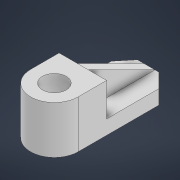
# Autodesk Inventor part: Pieza de práctica 4
Saved by Autodesk Inventor 2022 (Build 260153000, 153)
## iProperties
Created: 2022-06-27
Part Number: Pieza de práctica 4
Material: Genérico
Document SubType Name: Modeling
Designer: aleon
Density: 1 g/cm^3
Appearance: Valor por defecto
Author: aleon
Autodesk Inventor part; units mm, degrees
ref_plane "YZ Plane" through (0, 0, 0) normal (1, 0, 0) x (0, 1, 0)
ref_plane "XZ Plane" through (0, 0, 0) normal (0, 1, 0) x (-1, 0, 0)
ref_plane "XY Plane" through (0, 0, 0) normal (0, 0, 1) x (1, 0, 0)
sketch "Boceto1" plane through (0, 0, 0) normal (0, 1, 0) x (-1, 0, 0)
  circle A0 centre (0, 0) radius 7.5
  arc A1 (15, 0) -> (-15, 0) centre (0, 0) ccw
  line L0 (-15, 0) -> (-15, -51)
  line L1 (-15, -51) -> (-6, -60)
  line L2 (-6, -60) -> (7.5, -60)
  line L3 (7.5, -60) -> (15, -51)
  line L4 (15, -51) -> (15, 0)
  line L5 (15, -18) -> (-15, -18)
  dimension "d0" = 15
  dimension "d1" = 30
  dimension "d2" = 60
  dimension "d3" = 18
  dimension "d4" = 9
  dimension "d5" = 9
  constraints: 12 end point, 2 centre point, 2 coincident, 2 perpendicular, 2 point on circle, 2 point on line, 2 tangent, 1 horizontal alignment, 1 parallel, 1 vertical
  measures "d0" diameter of A0
  measures "d1" diameter of A1
  measures "d2" vertical distance of L1.end L0.start
  measures "d3" distance from line of L5 L4.end
  measures "d4" horizontal distance of L1.end L0.end
  measures "d5" vertical distance of L1.end L3.end
extrude "Extrusión1" add sketch "Boceto1" along normal blind 30 contours L4 L5 L0 A1
extrude "Extrusión2" add sketch "Boceto1" along normal blind 9 contours L4 L3 L2 L1 L0 L5
sketch "Boceto2" plane through (0, 0, 0) normal (1, 0, 0) x (0, 1, 0)
  line L0 (30, -18) -> (30, 0) projected
  line L1 (9, -60) -> (9, -51) projected
  line L2 (30, -18) -> (9, -60)
  line L3 (9, -60) -> (9, -18)
  line L4 (9, -18) -> (30, -18)
  point P0 (0, 0)
  constraints: 6 end point, 1 collinear, 1 perpendicular
extrude "Extrusión3" add sketch "Boceto2" along normal mid plane 7
